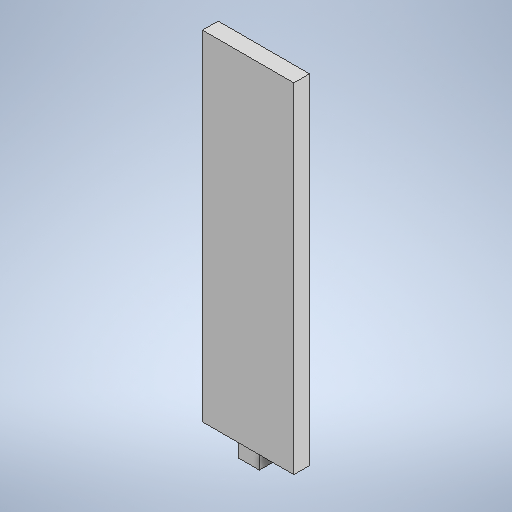
# Autodesk Inventor part: carcasa_piezasRadio_3.0
Saved by Autodesk Inventor 2025.3 (Build 293356030, 356C)
## iProperties
Created: 2025-09-04
Part Number: carcasa_piezasRadio_3.0
Material: Generic
Document SubType Name: Modeling
Designer: brene
Density: 1 g/cm^3
Appearance: Default
Author: brene
Autodesk Inventor part; units mm, degrees
ref_plane "YZ Plane" through (0, 0, 0) normal (1, 0, 0) x (0, 1, 0)
ref_plane "XZ Plane" through (0, 0, 0) normal (0, 1, 0) x (-1, 0, 0)
ref_plane "XY Plane" through (0, 0, 0) normal (0, 0, 1) x (1, 0, 0)
sketch "Sketch3" plane through (0, 0, 0) normal (0, 0, 1) x (1, 0, 0)
  line L0 (0, 0) -> (17.5, 0)
  line L1 (17.5, 0) -> (17.5, 65)
  line L2 (17.5, 65) -> (0, 65)
  line L3 (0, 65) -> (0, 0)
  dimension "d0" = 17.5
  dimension "d1" = 65
  dimension "d2" = 17.5
  constraints: 8 end point, 2 perpendicular, 1 horizontal
  measures "d0" distance of L0.start L0.end
  measures "d1" distance of L0.end L1.end
  measures "d2" distance of L1.end L2.end
extrude "Extrusion1" add sketch "Sketch3" along normal blind 3
sketch "Sketch4" plane through (0, 0, 0) normal (0, -1, 0) x (1, 0, 0)
  line L0 (0, 0) -> (0, 3) projected
  line L1 (0, 1.5) -> (17.5, 1.5)
  line L2 (17.5, 0) -> (17.5, 3) projected
  line L3 (17.5, 3) -> (0, 3) projected
  line L4 (8.75, 3) -> (8.75, 0)
  line L5 (17.5, 0) -> (0, 0) projected
  line L6 (8.75, 1.5) -> (6.75, 1.5)
  line L7 (6.75, 1.5) -> (6.75, 2.85)
  line L8 (8.75, 1.5) -> (10.75, 1.5)
  line L9 (10.75, 1.5) -> (10.75, 0.15)
  line L10 (6.75, 2.85) -> (10.75, 2.85)
  line L11 (10.75, 2.85) -> (10.75, 0.15)
  line L12 (10.75, 0.15) -> (6.75, 0.15)
  line L13 (6.75, 0.15) -> (6.75, 2.85)
  dimension "d5" = 2
  dimension "d6" = 1.35
  dimension "d7" = 2
  dimension "d8" = 1.35
  constraints: 20 end point, 5 midpoint, 3 perpendicular, 2 parallel, 2 point on line, 1 horizontal
  measures "d5" distance of L6.start L6.end
  measures "d6" distance of L6.end L7.end
  measures "d7" distance of L6.start L8.end
  measures "d8" distance of L8.end L9.end
extrude "Extrusion2" add sketch "Sketch4" along normal blind 2.7 contours L7 L10 L4 L1 | L1 L4 L12 L13 | L4 L1 L9 L12 | L4 L10 L11 L1
body "Solid1"
